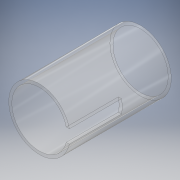
# Autodesk Inventor part: cylindre-lanceur
Saved by Autodesk Inventor 2017 (Build 210142000, 142)
## iProperties
Created: 2018-01-27
Part Number: cylindre-lanceur
Material: Generic
Document SubType Name: Modeling
Designer: franc
Density: 1 g/cm^3
Appearance: Polycarbonate - Transparent
Author: franc
Autodesk Inventor part; units mm, degrees
ref_plane "XZ Plane" through (0, 0, 0) normal (0, 1, 0) x (-1, 0, 0)
ref_plane "XY Plane" through (0, 0, 0) normal (0, 0, 1) x (1, 0, 0)
sketch "Esquisse1" plane through (0, 0, 0) normal (0, 1, 0) x (-1, 0, 0)
  circle A0 centre (0, 0) radius 27
  circle A1 centre (0, 0) radius 30
  dimension "d0" = 60
  dimension "d1" = 54
  constraints: 2 centre point, 2 coincident
  measures "d0" diameter of A1
  measures "d1" diameter of A0
extrude "Extrusion1" add sketch "Esquisse1" along normal blind 125
ref_plane "Plan de construction1" through (30, 0, 0) normal (1, 0, 0) x (0, 1, 0)
sketch "Esquisse2" plane through (30, 0, 0) normal (1, 0, 0) x (0, 1, 0)
  line L0 (77, 6.5) -> (26, 6.5)
  line L1 (26, 6.5) -> (26, -6.5)
  line L2 (26, -6.5) -> (77, -6.5)
  line L3 (77, -6.5) -> (77, 6.5)
  line L4 (0, -27) -> (0, 27) projected
  line L5 (-25, 0) -> (150, 0) projected
  point P0 (0, 0)
  dimension "d5" = 26
  dimension "d6" = 51
  dimension "d7" = 13
  dimension "d8" = 6.5
  constraints: 8 end point, 2 parallel, 1 horizontal, 1 perpendicular
  measures "d5" distance between parallel lines of L4 L1
  measures "d6" distance of L0.start L0.end
  measures "d7" distance of L2.end L0.start
  measures "d8" distance between parallel lines of L5 L0
extrude "Extrusion2" cut sketch "Esquisse2" against normal blind 10
sketch "Esquisse3" plane through (0, 0, 0) normal (0, -1, 0) x (1, 0, 0)
  circle A0 centre (0, 0) radius 27
  circle A1 centre (0, 0) radius 30
  dimension "d11" = 54
  dimension "d12" = 60
  constraints: 2 centre point, 2 coincident
  measures "d11" diameter of A0
  measures "d12" diameter of A1
extrude "Extrusion3" cut sketch "Esquisse3" against normal blind 26
